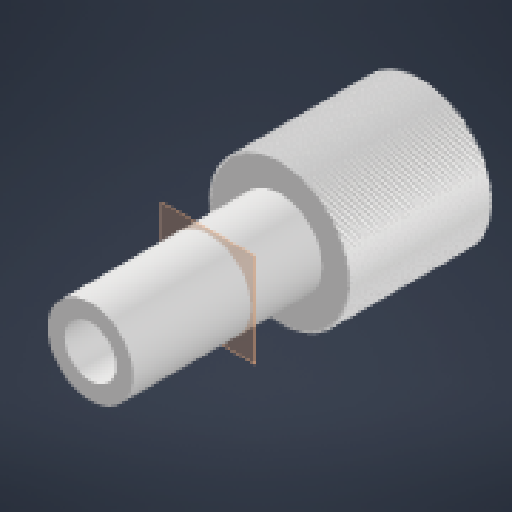
# Autodesk Inventor part: Dial2
Saved by Autodesk Inventor 2027 (Build 310192000, 192)
## iProperties
Created: 2026-03-03
Part Number: Dial2
Material: Generic
Document SubType Name: Modeling
Designer: kjedr
Density: 1 g/cm^3
Appearance: Default
Author: kjedr
Autodesk Inventor part; units mm, degrees
ref_plane "YZ Plane" through (0, 0, 0) normal (1, 0, 0) x (0, 1, 0)
ref_plane "XZ Plane" through (0, 0, 0) normal (0, 1, 0) x (-1, 0, 0)
ref_plane "XY Plane" through (0, 0, 0) normal (0, 0, 1) x (1, 0, 0)
sketch "Sketch1" plane through (0, 0, 0) normal (0, 0, 1) x (1, 0, 0)
  circle A0 centre (0, 0) radius 9.525
  dimension "d0" = 19.05
  constraints: 1 centre point, 1 coincident
  measures "d0" diameter of A0
extrude "Extrusion1" add sketch "Sketch1" along normal blind 3.81
sketch "Sketch2" plane through (0, 0, 3.81) normal (0, 0, 1) x (1, 0, 0)
  circle A0 centre (0, 0) radius 5.715
  dimension "d3" = 11.43
  constraints: 1 centre point, 1 coincident
  measures "d3" diameter of A0
extrude "Extrusion3" add sketch "Sketch2" along normal blind 10.16
sketch "Sketch4" plane through (0, 0, 0) normal (0, 0, -1) x (-1, 0, 0)
  circle A0 centre (0, 0) radius 9.525 projected
  line L0 (0, 9.525) -> (0, 9.144) construction
  line L1 (0, 9.525) -> (0.1905, 9.525) construction
  line L2 (0, 9.525) -> (-0.1905, 9.525) construction
  line L3 (0, 9.525) -> (0.1905, 9.525) construction
  line L4 (-0.1905, 9.525) -> (0, 9.144)
  line L5 (0.1905, 9.525) -> (0, 9.144)
  point P0 (0.1896, 9.5231)
  point P1 (-0.1896, 9.5231)
  dimension "d15" = 0.381
  dimension "d16" = 0.1905
  dimension "d17" = 0.1905
  dimension "d18" = 180
  constraints: 12 end point, 5 horizontal, 1 coincident, 1 collinear, 1 vertical, 2 other
  measures "d15" distance of L0.start L0.end
  measures "d16" distance of L0.start L1.end
  measures "d17" distance of L0.start L2.end
  measures "d18" angle of L2 L3
extrude "Extrusion4" cut sketch "Sketch4" against normal through all contours L5 L4 A0 picked at (0, 9.3979)
pattern_circular "Circular Pattern1" count 150 over 360 about axis through (0, 0, -10) along (0, 0, 1) of "Extrusion4"
sketch "Sketch5" plane through (0, 0, 13.97) normal (0, 0, 1) x (1, 0, 0)
  circle A0 centre (0, 0) radius 3.429
  line L0 (1.143, 3.2329) -> (1.143, -3.2329)
  dimension "d33" = 6.858
  dimension "d34" = 1.143
  constraints: 2 end point, 2 point on circle, 1 centre point, 1 coincident, 1 vertical
  measures "d33" diameter of A0
  measures "d34" distance from line of point (0, 0) L0
extrude "Extrusion5" cut sketch "Sketch5" against normal blind 25.4 contours A0 L0 picked at (2.6203, -0.1828)
extrude "Extrusion6" cut sketch "Sketch5" against normal blind 12.7 contours L0 A0 picked at (-0.7017, -0.9282)
body "Solid1"
